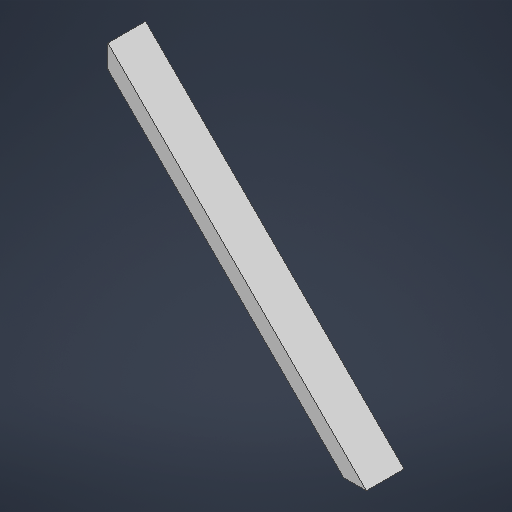
# Autodesk Inventor part: S_2x4x33.941
Saved by Autodesk Inventor 2026 (Build 300175000, 175)
## iProperties
Created: 2025-09-04
Part Number: S_2x4x33.941
Material: Generic
Document SubType Name: Modeling
Designer: trott
Density: 1 g/cm^3
Appearance: Default
Author: trott
Autodesk Inventor part; units mm, degrees
ref_plane "YZ Plane" through (0, 0, 0) normal (1, 0, 0) x (0, 1, 0)
ref_plane "XZ Plane" through (0, 0, 0) normal (0, 1, 0) x (-1, 0, 0)
ref_plane "XY Plane" through (0, 0, 0) normal (0, 0, 1) x (1, 0, 0)
sketch "Sketch1" plane through (0, 0, 0) normal (0, 0, 1) x (1, 0, 0)
  line L0 (0, 0) -> (0, 609.6)
  line L1 (0, 0) -> (860.5185, 0)
  line L2 (0, 609.6) -> (265.6478, 609.6)
  line L3 (304.8, 609.6) -> (914.4, 0)
  line L4 (304.8, 609.6) -> (304.8, 555.7185)
  line L5 (0, 609.6) -> (0, 682.9906)
  line L6 (0, 682.9906) -> (0, 1732.1998)
  line L7 (0, 1902.1906) -> (304.8, 609.6)
  line L8 (304.8, 609.6) -> (267.717, 600.8556)
  line L9 (304.8, 609.6) -> (277.8592, 582.6592)
  line L10 (914.4, 0) -> (887.4592, -26.9408)
  line L11 (277.8592, 582.6592) -> (304.8, 555.7185)
  line L12 (0, 1902.1906) -> (-38.1, 1893.2064)
  line L13 (-38.1, 1893.2064) -> (0, 1732.1998)
  line L14 (265.6478, 609.6) -> (267.717, 600.8556)
  line L15 (265.6478, 609.6) -> (304.8, 609.6)
  line L16 (304.8, 555.7185) -> (304.8, 0)
  line L17 (304.8, 555.7185) -> (860.5185, 0)
  line L18 (860.5185, 0) -> (914.4, 0)
  line L19 (860.5185, 0) -> (887.4592, -26.9408)
  line L20 (0, 1732.1998) -> (265.6478, 609.6)
  line L21 (0, 1732.1998) -> (0, 1902.1906)
  dimension "d0" = 609.6
  dimension "d1" = 914.4
  dimension "d2" = 304.8
  dimension "d3" = 1219.2
  dimension "d5" = 38.1
  dimension "d6" = 38.1
  dimension "d7" = 90
  dimension "d8" = 90
  dimension "d9" = 38.1
  dimension "d10" = 90
  dimension "d13" = 38.1
  constraints: 44 end point, 4 horizontal, 4 perpendicular, 2 point on line, 1 vertical
  measures "d0" distance of L0.start L0.end
  measures "d1" distance of L0.start L3.end
  measures "d2" distance of L0.end L3.start
  measures "d3" distance of L5.end L7.start
  measures "d5" distance of L3.start L8.end
  measures "d6" distance of L3.start L9.end
  measures "d7" angle of L3 L9
  measures "d8" angle of L7 L8
  measures "d9" distance of L10.start L10.end
  measures "d10" angle of L3 L10
  measures "d13" horizontal distance of L7.start L12.end
extrude "Extrusion1" add sketch "Sketch1" along normal blind 88.9 contours L17 L4 L3 L18
body "Solid1"
